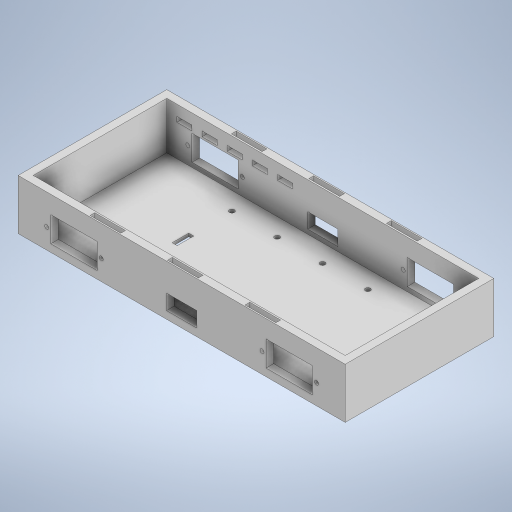
# Autodesk Inventor part: cuerpo3
Saved by Autodesk Inventor 2024.3 (Build 283343000, 343)
## iProperties
Created: 2025-10-08
Part Number: cuerpo3
Material: Generic
Document SubType Name: Modeling
Designer: jscme
Density: 1 g/cm^3
Appearance: Default
Author: jscme
Autodesk Inventor part; units mm, degrees
ref_plane "YZ Plane" through (0, 0, 0) normal (1, 0, 0) x (0, 1, 0)
ref_plane "XZ Plane" through (0, 0, 0) normal (0, 1, 0) x (-1, 0, 0)
sketch "Sketch1" plane through (0, 0, 0) normal (0, 1, 0) x (-1, 0, 0)
  line L0 (82.5, 37.5) -> (-82.5, 37.5)
  line L1 (-82.5, 37.5) -> (-82.5, -37.5)
  line L2 (-82.5, -37.5) -> (82.5, -37.5)
  line L3 (82.5, -37.5) -> (82.5, 37.5)
  point P0 (0, 0)
  point P1 (82.5, 0)
  point P2 (0, -37.5)
  dimension "d0" = 165
  dimension "d1" = 75
  constraints: 8 end point, 2 midpoint, 2 parallel, 1 horizontal, 1 horizontal alignment, 1 perpendicular, 1 vertical alignment
  measures "d0" distance of L1.end L2.end
  measures "d1" distance of L2.end L0.start
extrude "Extrusion1" add sketch "Sketch1" along normal blind 25.4
sketch "Sketch2" plane through (-82.5, 0, 37.5) normal (0, 0, 1) x (1, 0, 0)
  line L0 (39.878, 16.51) -> (16.51, 16.51)
  line L1 (39.878, 3.81) -> (39.878, 16.51)
  line L2 (16.51, 3.81) -> (39.878, 3.81)
  line L3 (16.51, 16.51) -> (16.51, 3.81)
  circle A0 centre (14.4272, 10.16) radius 1.016
  circle A1 centre (41.9608, 10.16) radius 1.016
  line L4 (0, 0) -> (165, 0) projected
  line L5 (0, 0) -> (0, 25.4) projected
  line L6 (148.49, 16.51) -> (125.122, 16.51)
  circle A2 centre (150.5728, 10.16) radius 1.016
  line L7 (148.49, 3.81) -> (148.49, 16.51)
  line L8 (125.122, 3.81) -> (148.49, 3.81)
  line L9 (125.122, 16.51) -> (125.122, 3.81)
  circle A3 centre (123.0392, 10.16) radius 1.016
  line L10 (165, 0) -> (165, 25.4) projected
  line L11 (74.88, 11.43) -> (90.12, 11.43)
  line L12 (90.12, 11.43) -> (90.12, 3.81)
  line L13 (90.12, 3.81) -> (74.88, 3.81)
  line L14 (74.88, 3.81) -> (74.88, 11.43)
  point P0 (82.5, 0)
  point P1 (16.51, 10.16)
  point P2 (39.878, 10.16)
  point P3 (0, 12.7)
  point P4 (125.122, 10.16)
  point P5 (82.5, 11.43)
  point P6 (82.5, 0)
  point P7 (74.88, 7.62)
  point P8 (148.49, 10.16)
  point P9 (90.12, 7.62)
  dimension "d4" = 12.7
  dimension "d5" = 23.368
  dimension "d6" = 2.032
  dimension "d7" = 2.032
  dimension "d8" = 2.0828
  dimension "d9" = 2.0828
  dimension "d11" = 16.51
  dimension "d12" = 12.7
  dimension "d13" = 23.368
  dimension "d14" = 2.032
  dimension "d15" = 2.032
  dimension "d16" = 2.0828
  dimension "d17" = 2.0828
  dimension "d18" = 16.51
  dimension "d19" = 15.24
  dimension "d20" = 7.62
  dimension "d55" = 10.16
  dimension "d56" = 10.16
  dimension "d58" = 7.62
  constraints: 24 end point, 9 midpoint, 6 parallel, 4 centre point, 4 horizontal alignment, 3 horizontal, 3 perpendicular, 1 vertical alignment
  measures "d4" distance of L1.start L0.start
  measures "d5" distance of L2.start L1.start
  measures "d6" diameter of A1
  measures "d7" diameter of A0
  measures "d8" distance from line of A1.centre L1
  measures "d9" distance from line of L3 A0.centre
  measures "d11" distance from line of point (0, 12.7) L3
  measures "d12" distance of L7.start L6.start
  measures "d13" distance of L8.start L7.start
  measures "d14" diameter of A2
  measures "d15" diameter of A3
  measures "d16" distance from line of A2.centre L7
  measures "d17" distance from line of L9 A3.centre
  measures "d18" distance between parallel lines of L10 L7
  measures "d19" distance between parallel lines of L14 L12
  measures "d20" distance between parallel lines of L13 L11
  measures "d55" distance from line of L4 point (39.878, 10.16)
  measures "d56" distance from line of L4 point (148.49, 10.16)
  measures "d58" distance from line of L4 point (90.12, 7.62)
extrude "Extrusion2" cut sketch "Sketch2" against normal blind 100.0125
sketch "Sketch3" plane through (0, 25.4, 0) normal (0, 1, 0) x (1, 0, 0)
  line L0 (-78.69, 33.69) -> (78.69, 33.69)
  line L1 (78.69, 33.69) -> (78.69, -33.69)
  line L2 (78.69, -33.69) -> (-78.69, -33.69)
  line L3 (-78.69, -33.69) -> (-78.69, 33.69)
  line L4 (82.5, -37.5) -> (82.5, 37.5) projected
  line L5 (-82.5, 37.5) -> (-82.5, -37.5) projected
  line L6 (82.5, 37.5) -> (-82.5, 37.5) projected
  line L7 (-82.5, -37.5) -> (82.5, -37.5) projected
  point P0 (0, 0)
  dimension "d25" = 3.81
  dimension "d26" = 3.81
  dimension "d27" = 3.81
  dimension "d28" = 3.81
  constraints: 8 end point, 2 parallel, 1 horizontal, 1 perpendicular
  measures "d25" distance between parallel lines of L4 L1
  measures "d26" distance between parallel lines of L5 L3
  measures "d27" distance between parallel lines of L6 L0
  measures "d28" distance between parallel lines of L7 L2
extrude "Extrusion3" cut sketch "Sketch3" against normal blind 23.8125 contours L0 L1 L2 L3
sketch "Sketch4" plane through (0, 1.5875, 0) normal (0, 1, 0) x (1, 0, 0)
  circle A0 centre (31.7833, 24.6457) radius 1.27
  line L0 (-42.5, 20.5817) -> (42.5, 20.5817)
  circle A1 centre (8.9233, 24.6457) radius 1.27
  circle A2 centre (-13.9367, 24.6457) radius 1.27
  circle A3 centre (-36.7967, 24.6457) radius 1.27
  line L1 (67.3028, 0) -> (-67.3028, 0)
  circle A4 centre (31.7833, -24.6457) radius 1.27
  circle A5 centre (8.9233, -24.6457) radius 1.27
  circle A6 centre (-13.9367, -24.6457) radius 1.27
  circle A7 centre (-36.7967, -24.6457) radius 1.27
  line L2 (78.69, 33.69) -> (78.69, -33.69) projected
  line L3 (-38.0667, -4.2532) -> (-35.5267, -4.2532)
  line L4 (-35.5267, -4.2532) -> (-35.5267, 4.1493)
  line L5 (-35.5267, 4.1493) -> (-38.0667, 4.1493)
  line L6 (-38.0667, 4.1493) -> (-38.0667, -4.2532)
  point P0 (0, 0)
  point P1 (-11.4746, -1.9183)
  point P2 (78.69, 0)
  point P3 (0, 0)
  point P4 (0, 20.5817)
  point P5 (-36.7967, -4.2532)
  dimension "d35" = 2.54
  dimension "d36" = 4.064
  dimension "d37" = 22.86
  dimension "d159" = 20.3925
  dimension "d160" = 49.2914
  constraints: 12 end point, 8 centre point, 4 midpoint, 4 symmetric about line, 3 horizontal, 2 parallel, 1 coincident, 1 horizontal alignment, 1 perpendicular, 1 vertical alignment, 10 other
  measures "d35" diameter of A0
  measures "d36" distance from line of L0 A0.centre
  measures "d37" distance of A0.centre A1.centre
  measures "d159" distance of point (-36.797, -4.253) A7.centre
  measures "d160" distance of A3.centre A7.centre
extrude "Extrusion4" cut sketch "Sketch4" against normal blind 22.225
ref_plane "Work Plane2" through (0, 19.05, 0) normal (0, 1, 0) x (1, 0, 0)
sketch "Sketch9" plane through (0, 25.4, 0) normal (0, 1, 0) x (1, 0, 0)
  line L0 (-46.8649, 36.8624) -> (-31.3709, 36.8624)
  line L1 (-31.3709, 36.8624) -> (-31.3709, 34.452)
  line L2 (-31.3709, 34.452) -> (-46.8649, 34.452)
  line L3 (-46.8649, 34.452) -> (-46.8649, 36.8624)
  line L4 (31.3709, 36.8624) -> (46.8649, 36.8624)
  line L5 (46.8649, 36.8624) -> (46.8649, 34.452)
  line L6 (46.8649, 34.452) -> (31.3709, 34.452)
  line L7 (31.3709, 34.452) -> (31.3709, 36.8624)
  line L8 (-7.7489, 36.8624) -> (7.7489, 36.8624)
  line L9 (7.7489, 36.8624) -> (7.7489, 34.452)
  line L10 (7.7489, 34.452) -> (-7.7489, 34.452)
  line L11 (-7.7489, 34.452) -> (-7.7489, 36.8624)
  line L12 (82.5, -37.5) -> (82.5, 37.5) projected
  line L13 (-82.5, 37.5) -> (-82.5, -37.5) projected
  line L14 (-67.8534, 0) -> (73.4776, 0)
  line L15 (-46.8649, -36.8624) -> (-31.3709, -36.8624)
  line L16 (-31.3709, -36.8624) -> (-31.3709, -34.452)
  line L17 (-31.3709, -34.452) -> (-46.8649, -34.452)
  line L18 (-46.8649, -34.452) -> (-46.8649, -36.8624)
  line L19 (31.3709, -36.8624) -> (46.8649, -36.8624)
  line L20 (46.8649, -36.8624) -> (46.8649, -34.452)
  line L21 (46.8649, -34.452) -> (31.3709, -34.452)
  line L22 (31.3709, -34.452) -> (31.3709, -36.8624)
  line L23 (-7.7489, -36.8624) -> (7.7489, -36.8624)
  line L24 (7.7489, -36.8624) -> (7.7489, -34.452)
  line L25 (7.7489, -34.452) -> (-7.7489, -34.452)
  line L26 (-7.7489, -34.452) -> (-7.7489, -36.8624)
  line L27 (-78.69, 33.69) -> (78.69, 33.69) projected
  point P0 (0, 0)
  point P1 (-31.3709, 35.6572)
  point P2 (31.3709, 35.6572)
  point P3 (-7.7489, 35.6572)
  point P4 (7.7489, 35.6572)
  point P5 (0, 34.452)
  dimension "d59" = 2.4104
  dimension "d60" = 2.4104
  dimension "d61" = 2.4104
  dimension "d62" = 23.622
  dimension "d63" = 23.622
  dimension "d64" = 15.4979
  dimension "d65" = 15.494
  dimension "d66" = 15.494
  dimension "d85" = 0.762
  constraints: 50 end point, 12 symmetric about line, 6 parallel, 5 midpoint, 4 horizontal, 3 perpendicular, 2 horizontal alignment, 1 vertical alignment
  measures "d59" distance between parallel lines of L2 L0
  measures "d60" distance between parallel lines of L6 L4
  measures "d61" distance between parallel lines of L10 L8
  measures "d62" distance between parallel lines of L1 L11
  measures "d63" distance between parallel lines of L7 L9
  measures "d64" distance of L9.end L10.end
  measures "d65" distance of L5.end L6.end
  measures "d66" distance of L1.end L2.end
  measures "d85" distance between parallel lines of L27 L10
extrude "Extrusion6" cut sketch "Sketch9" against normal blind 6.35
sketch "Sketch12" plane through (-78.69, 25.4, -33.69) normal (0, 0, 1) x (1, 0, 0)
  line L0 (5.08, -5.334) -> (12.7, -5.334)
  line L1 (12.7, -5.334) -> (12.7, -7.874)
  line L2 (12.7, -7.874) -> (5.08, -7.874)
  line L3 (5.08, -7.874) -> (5.08, -5.334)
  line L4 (0, 0) -> (157.38, 0) projected
  line L5 (0, 0) -> (0, -23.8125) projected
  line L6 (17.78, -5.334) -> (25.4, -5.334)
  line L7 (25.4, -5.334) -> (25.4, -7.874)
  line L8 (25.4, -7.874) -> (17.78, -7.874)
  line L9 (17.78, -7.874) -> (17.78, -5.334)
  line L10 (30.48, -5.334) -> (38.1, -5.334)
  line L11 (38.1, -5.334) -> (38.1, -7.874)
  line L12 (38.1, -7.874) -> (30.48, -7.874)
  line L13 (30.48, -7.874) -> (30.48, -5.334)
  line L14 (43.18, -5.334) -> (50.8, -5.334)
  line L15 (50.8, -5.334) -> (50.8, -7.874)
  line L16 (50.8, -7.874) -> (43.18, -7.874)
  line L17 (43.18, -7.874) -> (43.18, -5.334)
  line L18 (55.88, -5.334) -> (63.5, -5.334)
  line L19 (63.5, -5.334) -> (63.5, -7.874)
  line L20 (63.5, -7.874) -> (55.88, -7.874)
  line L21 (55.88, -7.874) -> (55.88, -5.334)
  point P0 (78.69, -25.4)
  dimension "d123" = 2.54
  dimension "d124" = 7.62
  dimension "d125" = 5.334
  dimension "d126" = 5.08
  dimension "d127" = 7.62
  dimension "d128" = 2.54
  dimension "d129" = 5.334
  dimension "d130" = 5.08
  dimension "d131" = 7.62
  dimension "d132" = 2.54
  dimension "d133" = 5.334
  dimension "d134" = 5.08
  dimension "d135" = 7.62
  dimension "d136" = 2.54
  dimension "d137" = 5.334
  dimension "d138" = 5.08
  dimension "d139" = 7.62
  dimension "d140" = 2.54
  dimension "d141" = 5.334
  dimension "d142" = 5.08
  constraints: 40 end point, 10 parallel, 5 horizontal, 5 perpendicular
  measures "d123" distance between parallel lines of L2 L0
  measures "d124" distance of L1.end L2.end
  measures "d125" distance between parallel lines of L4 L0
  measures "d126" distance between parallel lines of L5 L3
  measures "d127" distance of L6.start L6.end
  measures "d128" distance of L8.end L6.start
  measures "d129" distance between parallel lines of L4 L6
  measures "d130" distance between parallel lines of L1 L9
  measures "d131" distance of L11.end L12.end
  measures "d132" distance of L12.end L10.start
  measures "d133" distance between parallel lines of L4 L10
  measures "d134" distance between parallel lines of L7 L13
  measures "d135" distance of L15.end L16.end
  measures "d136" distance of L16.end L14.start
  measures "d137" distance between parallel lines of L4 L14
  measures "d138" distance between parallel lines of L11 L17
  measures "d139" distance of L19.end L20.end
  measures "d140" distance of L20.end L18.start
  measures "d141" distance between parallel lines of L4 L18
  measures "d142" distance between parallel lines of L15 L21
extrude "Extrusion9" cut sketch "Sketch12" against normal blind 5.715
body "Solid1"
